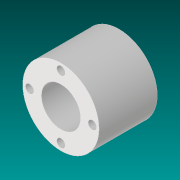
# Autodesk Inventor part: 轉接版
Saved by Autodesk Inventor 2020 (Build 240168000, 168)
## iProperties
Created: 2023-03-07
Part Number: 轉接版
Material: 一般
Document SubType Name: Modeling
Designer: ASUS
Density: 1 g/cm^3
Appearance: 預設
Author: ASUS
Autodesk Inventor part; units mm, degrees
ref_plane "YZ Plane" through (0, 0, 0) normal (1, 0, 0) x (0, 1, 0)
ref_plane "XZ Plane" through (0, 0, 0) normal (0, 1, 0) x (-1, 0, 0)
ref_plane "XY Plane" through (0, 0, 0) normal (0, 0, 1) x (1, 0, 0)
sketch "草圖1" plane through (0, 0, 0) normal (0, 0, 1) x (1, 0, 0)
  line L0 (0, 27.58) -> (0, -27.58) construction
  line L1 (0, -27.58) -> (0, 27.58) construction
  line L2 (-27.58, 0) -> (27.58, 0) construction
  circle A0 centre (0, 0) radius 10
  circle A1 centre (0, 0) radius 16.179 construction
  circle A2 centre (0, 0) radius 19.7
  point P0 (16.179, 0)
  dimension "d1" = 32.358
  dimension "d0" = 20
  dimension "d2" = 39.4
  constraints: 3 coincident, 2 centre point, 1 horizontal alignment, 1 point on line, 2 other
  measures "d0" diameter of A0
  measures "d2" diameter of A2
extrude "擠出1" add sketch "草圖1" along normal blind 30
hole "孔1" at (16.179, 0, 0) direction (0, 0, 1) diameter 4.134 depth 61.1
pattern_circular "環形陣列1" count 4 over 360 about axis through (0, 0, 0) along (0, 0, 1) of "孔1"
